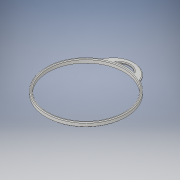
# Autodesk Inventor part: BladderHook
Saved by Autodesk Inventor 2017 (Build 210142000, 142)
## iProperties
Created: 2018-04-03
Part Number: BladderHook
Material: Generic
Document SubType Name: Modeling
Designer: jjaken
Density: 1 g/cm^3
Appearance: Default
Author: jjaken
Autodesk Inventor part; units mm, degrees
ref_plane "YZ Plane" through (0, 0, 0) normal (1, 0, 0) x (0, 1, 0)
ref_plane "XZ Plane" through (0, 0, 0) normal (0, 1, 0) x (-1, 0, 0)
ref_plane "XY Plane" through (0, 0, 0) normal (0, 0, 1) x (1, 0, 0)
sketch "Sketch1" plane through (0, 0, 0) normal (0, 1, 0) x (-1, 0, 0)
  circle A0 centre (0, 0) radius 52.5
  circle A1 centre (0, 0) radius 55.5
  dimension "d0" = 105
  dimension "d1" = 3
  constraints: 2 centre point, 2 coincident
  measures "d0" diameter of A0
  measures "d1" radial gap between concentric circles of A1 A0
extrude "Extrusion1" add sketch "Sketch1" along normal blind 6
sketch "Sketch2" plane through (0, 6, 0) normal (0, 1, 0) x (1, 0, 0)
  circle A0 centre (0, 0) radius 52.5
  circle A1 centre (0, 0) radius 55.5
  circle A2 centre (0, 0) radius 55.5 construction
  arc A3 (12.5, 54.074023) -> (-12.5, 54.074023) centre (0, 45.129327) ccw
  arc A4 (26.441888, 48.796276) -> (-26.441888, 48.796276) centre (0, 37.901631) ccw
  dimension "d4" = 6
  dimension "d5" = 25
  dimension "d6" = 5
  dimension "d7" = 52.88378
  constraints: 12 point on circle, 2 centre point, 2 vertical alignment
  measures "d5" distance of A1.start A1.end
  measures "d7" distance of A4.start A4.end
extrude "Extrusion2" add sketch "Sketch2" against normal blind 3 contours A1 A3 A4
fillet "Fillet1" radius 1 9 edges at (-47.6853, 6, -28.3965) (28.3965, 6, 47.6853) (52.5, 6, 0) (55.5, 0, 0) (52.5, 0, 0) (0, 6, -66.5) (0, 6, -60.5) (0, 3, -60.5) (0, 3, -66.5)
body "Solid1"
